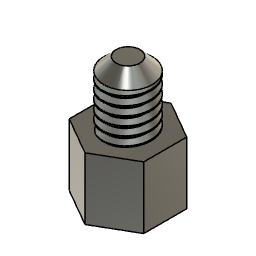
robot assembly v8 (Autodesk Fusion 360 archive; units mm, degrees)
design "screws"
Autodesk Fusion 360 part; units mm, degrees
sketch "Sketch1" plane through (0, 0, 0) normal (0, 0, 1) x (1, 0, 0)
  line L0 (0, 3.4641) -> (-3, 1.7321)
  line L1 (-3, 1.7321) -> (-3, -1.7321)
  line L2 (-3, -1.7321) -> (0, -3.4641)
  line L3 (0, -3.4641) -> (3, -1.7321)
  line L4 (3, -1.7321) -> (3, 1.7321)
  line L5 (3, 1.7321) -> (0, 3.4641)
  line L6 (0, 1.75) -> (0, 22.5)
  dimension "d1" = 3
  constraint coincident L0.start L6
  measures "d1" distance of origin L5
extrude "Extrude1" add sketch "Sketch1" along normal blind 5
sketch "Sketch2" plane through (0, 0, 5) normal (0, 0, 1) x (-1, 0, 0)
  line L0 (-3, -1.7321) -> (0, -3.4641)
  line L1 (0, -3.4641) -> (3, -1.7321)
  line L2 (3, -1.7321) -> (3, 1.7321)
  line L3 (3, 1.7321) -> (0, 3.4641)
  line L4 (0, 3.4641) -> (-3, 1.7321)
  line L5 (-3, 1.7321) -> (-3, -1.7321)
  circle A0 centre (0, 0) radius 2
  dimension "d4" = 4
  constraint coincident A0.centre origin
  measures "d4" diameter of A0
extrude "Extrude2" add sketch "Sketch2" along normal blind 5 contours A0
chamfer "Chamfer1" distance 1 angle 45 1 edges at (1.8647, 0.7232, 10)
thread "Thread1" "ISO Metric profile 4.0 M4x0.7 6g" major diameter 3.908 minor diameter 3.111 pitch 0.7 angle 60 modelled right hand crest width 0.1017 on face at (-1.9901, 0.1991, 7.6667) crest through (-1.954, 0, 4.825)
